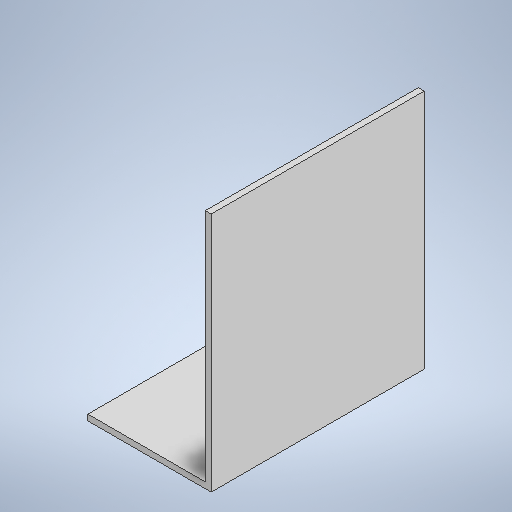
# Autodesk Inventor part: Box_Bottom
Saved by Autodesk Inventor 2025.1 (Build 291241020, 241B)
## iProperties
Created: 2025-03-03
Part Number: Box_Bottom
Material: Generic
Document SubType Name: Modeling
Designer: brett
Density: 1 g/cm^3
Appearance: Default
Author: brett
Autodesk Inventor part; units mm, degrees
ref_plane "YZ Plane" through (0, 0, 0) normal (1, 0, 0) x (0, 1, 0)
ref_plane "XZ Plane" through (0, 0, 0) normal (0, 1, 0) x (-1, 0, 0)
ref_plane "XY Plane" through (0, 0, 0) normal (0, 0, 1) x (1, 0, 0)
sketch "Sketch1" plane through (0, 0, 0) normal (0, 1, 0) x (-1, 0, 0)
  line L0 (0, 0) -> (106.68, 0)
  line L1 (106.68, 0) -> (106.68, -184.15)
  line L2 (106.68, -184.15) -> (0, -184.15)
  line L3 (0, -184.15) -> (0, 0)
  dimension "d0" = 184.15
  dimension "d1" = 106.68
  constraints: 8 end point, 2 parallel, 1 horizontal, 1 perpendicular
  measures "d0" distance of L0.end L1.end
  measures "d1" distance of L1.end L2.end
extrude "Extrusion1" add sketch "Sketch1" along normal blind 5.08
sketch "Sketch2" plane through (0, 5.08, 0) normal (0, 1, 0) x (1, 0, 0)
  line L0 (-5.08, 0) -> (-5.08, 184.15)
  line L1 (0, 0) -> (0, 184.15) projected
  line L2 (-5.08, 0) -> (0, 0)
  line L3 (0, 184.15) -> (-106.68, 184.15) projected
  line L4 (-5.08, 184.15) -> (0, 184.15)
  dimension "d4" = 5.08
  constraints: 7 end point, 2 horizontal, 1 point on line, 1 vertical
  measures "d4" distance between parallel lines of L1 L0
extrude "Extrusion2" add sketch "Sketch2" along normal blind 203.2
body "Solid1"
